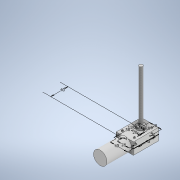
# Autodesk Inventor part: Motor_Gearbox
Saved by Autodesk Inventor 2020 (Build 240168000, 168)
## iProperties
Created: 2020-06-05
Part Number: Motor_Gearbox
Material: Generic
Document SubType Name: Modeling
Designer: jurre
Density: 1 g/cm^3
Appearance: Default
Author: jurre
Autodesk Inventor part; units mm, degrees
ref_plane "YZ Plane" through (0, 0, 0) normal (1, 0, 0) x (0, 1, 0)
ref_plane "XZ Plane" through (0, 0, 0) normal (0, 1, 0) x (-1, 0, 0)
ref_plane "XY Plane" through (0, 0, 0) normal (0, 0, 1) x (1, 0, 0)
sketch "Sketch1" plane through (0, 0, 0) normal (0, 1, 0) x (-1, 0, 0)
  line L0 (20, 37.5) -> (-20, 37.5)
  line L1 (-20, 37.5) -> (-20, -20.5)
  line L2 (-20, -20.5) -> (20, -20.5)
  line L3 (20, -20.5) -> (20, 37.5)
  circle A0 centre (14, -11.05) radius 2
  circle A1 centre (14, 28.95) radius 2
  circle A2 centre (-14, -11.05) radius 2
  circle A3 centre (-14, 28.95) radius 2
  circle A4 centre (0, 0) radius 9.4
  circle A5 centre (0, 0) radius 4
  dimension "d0" = 58
  dimension "d1" = 20.5
  dimension "d2" = 40
  dimension "d3" = 20
  dimension "d4" = 4
  dimension "d5" = 4
  dimension "d6" = 40
  dimension "d7" = 11.05
  dimension "d8" = 4
  dimension "d9" = 4
  dimension "d10" = 28
  dimension "d11" = 40
  dimension "d12" = 28
  dimension "d13" = 6
  dimension "d14" = 6
  dimension "d15" = 6
  dimension "d20" = 18.8
  dimension "d21" = 8
  constraints: 8 end point, 6 centre point, 2 coincident, 2 parallel, 1 horizontal, 1 perpendicular
  measures "d0" distance of L2.end L0.start
  measures "d1" distance from line of L2 point (0, 0)
  measures "d2" distance of L0.start L0.end
  measures "d3" distance from line of L3 point (0, 0)
  measures "d4" diameter of A0
  measures "d5" diameter of A1
  measures "d6" distance of A0.centre A1.centre
  measures "d7" vertical distance of A0.centre point (0, 0)
  measures "d8" diameter of A2
  measures "d9" diameter of A3
  measures "d10" distance of A2.centre A0.centre
  measures "d11" distance of A3.centre A2.centre
  measures "d12" distance of A3.centre A1.centre
  measures "d13" distance from line of L3 A0.centre
  measures "d14" distance from line of L1 A2.centre
  measures "d15" distance from line of L3 A1.centre
  measures "d20" diameter of A4
  measures "d21" diameter of A5
extrude "Extrusion1" add sketch "Sketch1" along normal mid plane 27 contours L3 L2 L1 L0 | A4 | A5
extrude "Extrusion2" add sketch "Sketch1" along normal mid plane 31 contours A0 | A1 | A2 | A3
extrude "Extrusion3" add sketch "Sketch1" along normal mid plane 36 contours A4
extrude "Extrusion4" add sketch "Sketch1" along normal blind 22 contours A5
sketch "Sketch2" plane through (-20, 13.5, 37.5) normal (0, 0, 1) x (1, 0, 0)
  circle A0 centre (20, -13.5) radius 15.5
  dimension "d26" = 31
  constraints: 1 centre point, 1 coincident
  measures "d26" diameter of A0
extrude "Extrusion5" add sketch "Sketch2" along normal blind 57
extrude "Extrusion6" add sketch "Sketch1" against normal blind 18 contours A5
hole "Hole1" at (-14, 0, 28.95) direction (0, 1, 0) diameter 3.242 end through all thread size "M4x0.7" class "6H" standard "ISO Metric profile"
hole "Hole2" at (14, 0, 28.95) direction (0, 1, 0) diameter 3.242 end through all thread size "M4x0.7" class "6H" standard "ISO Metric profile"
hole "Hole3" at (14, 0, -11.05) direction (0, 1, 0) diameter 3.242 end through all thread size "M4x0.7" class "6H" standard "ISO Metric profile"
hole "Hole4" at (-14, 0, -11.05) direction (0, 1, 0) diameter 3.242 end through all thread size "M4x0.7" class "6H" standard "ISO Metric profile"
sketch "Sketch5" plane through (0, 22, 0) normal (0, 1, 0) x (1, 0, 0)
  circle A0 centre (0, 0) radius 4 projected
extrude "Extrusion7" add sketch "Sketch5" along normal blind 116
thread "Thread1" size "M8x1.25" class "6g" standard "ANSI Metric M Profile" length 116 offset 4
body "Solid1"
